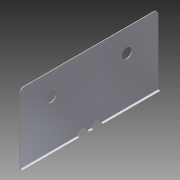
# Autodesk Inventor part: Fin_short
Saved by Autodesk Inventor 2015 (Build 190159000, 159)
## iProperties
Created: 2015-08-21
Part Number: Fin_short
Material: Aluminum 6061
Document SubType Name: Modeling
Designer: Kyle
Density: 2.7 g/cm^3
Appearance: Aluminum - Flat
Author: Kyle
Autodesk Inventor part; units mm, degrees
ref_plane "YZ Plane" through (0, 0, 0) normal (1, 0, 0) x (0, 1, 0)
ref_plane "XZ Plane" through (0, 0, 0) normal (0, 1, 0) x (-1, 0, 0)
ref_plane "XY Plane" through (0, 0, 0) normal (0, 0, 1) x (1, 0, 0)
sketch "Sketch1" plane through (0, 0, 0) normal (0, 0, 1) x (1, 0, 0)
  line L0 (0, 0) -> (1.8311, 0)
  line L1 (0, 0) -> (0, 45.085)
  line L2 (0.381, 45.085) -> (0.381, 0.381)
  line L3 (0.381, 0.381) -> (1.8311, 0.381)
  line L4 (1.8311, 0.381) -> (1.8311, 0)
  line L5 (0.381, 45.085) -> (0, 45.085)
  dimension "d0" = 1.8311
  dimension "d1" = 45.085
  dimension "d2" = 0.381
  constraints: 12 end point, 2 vertical, 1 horizontal, 1 perpendicular, 1 other
  measures "d0" distance of L0.start L0.end
  measures "d1" distance of L0.start L1.end
  measures "d2" distance between parallel lines of L1 L2
extrude "Extrusion1" add sketch "Sketch1" along normal blind 88.9
fillet "Fillet1" radius 2.54 2 edges at (0.1905, 45.085, 88.9) (0.1905, 45.085, 0)
sketch "Sketch2" plane through (0, 0, 0) normal (-1, 0, 0) x (0, 0, 1)
  line L0 (0, 0) -> (88.9, 0) projected
  circle A0 centre (40.005, 0) radius 3.175
  circle A1 centre (48.895, 0) radius 3.2307
  dimension "d6" = 6.35
  dimension "d7" = 8.89
  dimension "d8" = 40.005
  constraints: 2 centre point, 2 point on line
  measures "d6" diameter of A0
  measures "d7" distance of A0.centre A1.centre
  measures "d8" distance of L0.end A1.centre
extrude "Extrusion2" cut sketch "Sketch2" against normal blind 88.9
sketch "Sketch3" plane through (0, 0, 0) normal (-1, 0, 0) x (0, 0, 1)
  circle A0 centre (20.1258, 30.6113) radius 3.175
  circle A1 centre (68.8299, 30.6113) radius 3.175
  line L0 (88.9, 42.545) -> (88.9, 0) projected
  line L1 (0, 42.545) -> (0, 0) projected
  line L2 (2.54, 45.085) -> (86.36, 45.085) projected
  line L3 (68.8299, 30.6113) -> (48.9507, 0)
  line L4 (48.9507, 0) -> (88.9, 0)
  line L5 (20.1258, 30.6113) -> (40.005, 0)
  line L6 (0, 0.381) -> (36.8529, 0.381) projected
  line L7 (40.005, 0) -> (0, 0)
  point P0 (52.1257, 0)
  point P1 (36.83, 0)
  dimension "d11" = 6.35
  dimension "d12" = 6.35
  dimension "d19" = 3.175
  dimension "d20" = 3.175
  dimension "d21" = 36.4998
  dimension "d22" = 45.085
  dimension "d23" = 45.085
  dimension "d24" = 36.4998
  dimension "d25" = 57
  dimension "d26" = 57
  constraints: 8 end point, 2 centre point
  measures "d11" diameter of A0
  measures "d12" diameter of A1
  measures "d19" distance of L3.end point (52.126, 0)
  measures "d20" distance of point (36.83, 0) L5.end
  measures "d21" distance of L3.end L3.start
  measures "d22" distance from line of L2 L3.end
  measures "d23" distance from line of L2 L5.end
  measures "d24" distance of L5.start L5.end
  measures "d25" angle of L4 L3
  measures "d26" angle of L7 L5
extrude "Extrusion3" cut sketch "Sketch3" against normal blind 88.9
body "Solid1"
